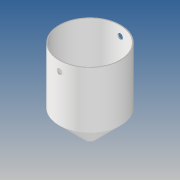
# Autodesk Inventor part: mineralisation
Saved by Autodesk Inventor 2020 (Build 240168000, 168)
## iProperties
Created: 2019-09-24
Part Number: mineralisation
Material: Generic
Document SubType Name: Modeling
Designer: a.komeijani
Density: 1 g/cm^3
Appearance: Default
Author: a.komeijani
Autodesk Inventor part; units mm, degrees
ref_plane "YZ Plane" through (0, 0, 0) normal (1, 0, 0) x (0, 1, 0)
ref_plane "XY Plane" through (0, 0, 0) normal (0, 0, 1) x (1, 0, 0)
sketch "Sketch1" plane through (0, 0, 0) normal (0, 0, 1) x (1, 0, 0)
  line L0 (542.1294, 0) -> (542.1294, -1000)
  line L1 (542.1294, -1000) -> (82.51, -1459.6194)
  line L2 (-7.8706, -896.0873) -> (-7.8706, -498.6597)
  line L3 (542.1294, 0) -> (542.1294, 0)
  line L4 (82.51, -1459.6194) -> (32.51, -1459.6194)
  line L5 (32.51, -1459.6194) -> (32.51, -1439.6194)
  line L6 (32.51, -1439.6194) -> (82.51, -1439.6194)
  line L7 (82.51, -1439.6194) -> (522.1294, -1000)
  line L8 (522.1294, -1000) -> (522.1294, 0)
  line L9 (522.1294, 0) -> (542.1294, 0)
  point P0 (0, 0)
  dimension "d0" = 1000
  dimension "d1" = 650
  dimension "d2" = 0
  dimension "d3" = 135
  dimension "d4" = 550
  dimension "d29" = 0
  dimension "d30" = 0
  dimension "d31" = 50
  dimension "d41" = 20
  constraints: 20 end point, 4 vertical, 2 horizontal, 2 parallel, 2 perpendicular, 1 coincident, 2 other
  measures "d0" distance of L0.start L0.end
  measures "d1" distance of L0.end L1.end
  measures "d2" distance of L1.end L4.start
  measures "d3" angle of L1 L0
  measures "d4" distance between parallel lines of L0 L2
  measures "d29" distance from line of point (0, 0) L3
  measures "d30" distance of L0.start L3.end
  measures "d31" distance of L4.start L4.end
  measures "d41" distance of L4.end L5.end
ref_plane "Work Plane6" through (-566.8771, -58.4878, 0) normal (0, -1, 0) x (1, 0, 0)
revolve "Revolution1" add sketch "Sketch1" angle 360 about axis through (-7.8706, -896.0873, 0) along (0, 1, 0)
sketch "Sketch41" plane through (0, 0, 0) normal (0, 0, 1) x (1, 0, 0)
  circle A0 centre (0, -166.4829) radius 50
  point P0 (0, 0)
  dimension "d143" = 100
  constraints: 1 centre point
  measures "d143" diameter of A0
extrude "Extrusion21" cut sketch "Sketch41" along normal mid plane 1200
sketch "Sketch19" plane through (0, 0, 0) normal (0, 0, 1) x (1, 0, 0)
  line L0 (32.51, -1559.6194) -> (-48.2512, -1559.6194) projected
  line L1 (-57.8706, -1559.6194) -> (42.1294, -1559.6194) projected
  circle A0 centre (-7.8706, -1559.6194) radius 50
  point P0 (0, 0)
  dimension "d68" = 100
  constraints: 1 centre point, 1 midpoint
  measures "d68" diameter of A0
sketch "Sketch20" plane through (-7.8706, -1559.6194, -650) normal (0, 0, -1) x (-1, 0, 0)
  circle A0 centre (0, 0) radius 40
  circle A1 centre (0, 0) radius 50 projected
  point P0 (-7.8706, 1559.6194)
  dimension "d71" = 80
  constraints: 1 centre point, 1 concentric
  measures "d71" diameter of A0
sketch "Sketch22" plane through (0, 0, 0) normal (1, 0, 0) x (0, 1, 0)
  line L0 (-1462.4815, 734.1369) -> (-140.2963, 734.1369)
  line L1 (-90.2963, 684.1369) -> (-90.2963, 550)
  arc A0 (-90.2963, 684.1369) -> (-140.2963, 734.1369) centre (-140.2963, 684.1369) ccw
  line L2 (-1558.0924, 663.4382) -> (-1558.0924, 643.3405)
  line L3 (-1509.6194, 650) -> (-1609.6194, 650) projected
  arc A1 (-1462.4815, 734.1369) -> (-1558.0924, 663.4382) centre (-1462.4815, 634.1369) ccw
  point P0 (0, 0)
  point P1 (-90.2963, 734.1369)
  dimension "d80" = 50
  constraints: 6 end point, 4 point on circle, 3 tangent, 2 centre point, 2 perpendicular, 2 point on line, 1 horizontal
  measures "d80" radius of A0
sketch "Sketch23" plane through (-7.8706, -1559.6194, 650) normal (0, 0, 1) x (1, 0, 0)
  circle A0 centre (0, 0) radius 40
  circle A1 centre (0, 0) radius 50
  point P0 (7.8706, 1559.6194)
  constraints: 2 centre point, 1 coincident
sketch "Sketch24" plane through (-7.8706, -88.7692, 550) normal (0, 0, -1) x (1, 0, 0)
  circle A0 centre (-5.435, 0.6448) radius 30.4902
  circle A1 centre (-5.435, 0.6448) radius 40
  point P0 (7.8706, -88.7692)
  dimension "d81" = 80
  constraints: 2 centre point, 1 coincident
  measures "d81" diameter of A1
sketch "Sketch26" plane through (0, 0, 0) normal (1, 0, 0) x (0, 1, 0)
  line L0 (-1459.6194, -722.3332) -> (-421.4562, -722.3332)
  arc A0 (-1559.6194, -622.3332) -> (-1459.6194, -722.3332) centre (-1459.6194, -622.3332) ccw
  line L1 (-1000, -530) -> (0, -530) projected
  line L2 (-421.4562, -722.3332) -> (-178.619, -722.3332)
  line L3 (-78.619, -622.3332) -> (-78.619, -548.782)
  arc A1 (-178.619, -722.3332) -> (-78.619, -622.3332) centre (-178.619, -622.3332) ccw
  point P0 (-1559.6194, -722.3332)
  dimension "d100" = 100
  dimension "d102" = 100
  constraints: 6 end point, 4 point on circle, 3 tangent, 2 centre point, 1 horizontal, 1 perpendicular, 1 point on line
  measures "d100" radius of A0
  measures "d102" radius of A1
sketch "Sketch29" plane through (0, 0, 0) normal (1, 0, 0) x (0, 1, 0)
  line L0 (-1509.6194, -650) -> (-1509.6194, 654.9469) projected
  line L1 (-1609.6194, -607.9379) -> (-1609.6194, 671.1566) projected
  line L2 (-1559.6194, 375.7234) -> (-1559.6194, 1195.913)
  point P0 (0, 0)
  constraints: 2 end point, 1 vertical
sketch "Sketch30" plane through (0, 0, 0) normal (0, 0, 1) x (1, 0, 0)
  circle A0 centre (-7.8706, -1559.5524) radius 50
  ellipse E0 centre (-7.8706, -1559.5524) end of major axis (42.1294, -1559.5524) minor radius 47.8054 (-57.8473, -1558.0924) -> (42.1061, -1558.0924) ccw projected
  point P0 (0, 0)
  dimension "d108" = 100
  constraints: 1 centre point, 2 other
  measures "d108" diameter of A0
sketch "Sketch31" plane through (-7.8706, -1559.5524, 820.1896) normal (0, 0, 1) x (1, 0, 0)
  arc A0 (-50, -0.0335) -> (50, -0.0335) centre (0, -0.067) ccw projected
  circle A1 centre (0, -0.067) radius 40
  point P0 (7.8706, 1559.5524)
  dimension "d2" = 0
  dimension "d111" = 80
  dimension "d114" = 130
  constraints: 2 end point, 2 other
sketch "Sketch35" plane through (0, 0, 0) normal (-0.6428, 0, -0.766) x (-0.766, 0, 0.6428)
  circle A0 centre (0, -300) radius 60
  circle A1 centre (0, -300) radius 50
  line L0 (-543.9708, 0) -> (556.0292, 0) projected
  point P0 (0, 0)
  dimension "d120" = 120
  dimension "d121" = 100
  dimension "d128" = 300
  constraints: 2 centre point, 1 concentric
  measures "d120" diameter of A0
  measures "d121" diameter of A1
  measures "d128" distance from line of A0.centre L0
sketch "Sketch36" plane through (-372.8168, -300, -444.3058) normal (-0.6428, 0, -0.766) x (-0.766, 0, 0.6428)
  circle A0 centre (0, 0) radius 50
  circle A1 centre (0, 0) radius 50 projected
  line L0 (-543.9708, 300) -> (556.0292, 300) projected
  point P0 (0, 300)
  dimension "d124" = 100
  dimension "d127" = 300
  constraints: 1 centre point, 1 concentric
  measures "d124" diameter of A0
  measures "d127" distance from line of A0.centre L0
sketch "Sketch37" plane through (0, 0, 0) normal (0, 1, 0) x (-1, 0, 0)
  circle A0 centre (7.8706, 735.664) radius 50
  circle A1 centre (7.8706, 735.664) radius 50 projected
  circle A2 centre (7.8706, 735.664) radius 40
  point P0 (0, 0)
  dimension "d129" = 100
  dimension "d130" = 80
  constraints: 2 centre point, 1 coincident, 1 concentric
  measures "d129" diameter of A0
  measures "d130" diameter of A2
sketch "Sketch38" plane through (-7.8706, 0, 735.664) normal (0, 1, 0) x (1, 0, 0)
  circle A0 centre (0, 0) radius 40 projected
  circle A1 centre (0, 0) radius 40
  point P0 (7.8706, 735.664)
  constraints: 1 centre point, 1 coincident
sketch "Sketch39" plane through (0, 0, 0) normal (0, 1, 0) x (-1, 0, 0)
  circle A0 centre (7.8706, -726.0843) radius 50
  ellipse E0 centre (7.8706, -726.0843) end of major axis (57.8706, -726.0843) minor radius 48.0483 projected
  point P0 (0, 0)
  point P1 (57.8706, -726.0843)
  dimension "d137" = 100
  constraints: 1 centre point, 1 horizontal alignment, 1 other
  measures "d137" diameter of A0
sketch "Sketch40" plane through (0, 0, 0) normal (0, 1, 0) x (1, 0, 0)
  circle A0 centre (-7.8706, 726.0843) radius 40
  ellipse E0 centre (-7.8706, 726.0843) end of major axis (-57.8706, 726.0843) minor radius 48.0483 projected
  point P0 (0, 0)
  dimension "d140" = 80
  constraints: 1 centre point, 2 other
  measures "d140" diameter of A0
sketch "Sketch25" plane through (-7.8706, -1559.6194, -650) normal (0, 0, -1) x (-1, 0, 0)
  circle A0 centre (0, 0) radius 40
  circle A1 centre (0, 0) radius 40 projected
  circle A2 centre (0, 0) radius 50
  constraints: 2 centre point, 1 coincident, 1 concentric
body "Solid3"
